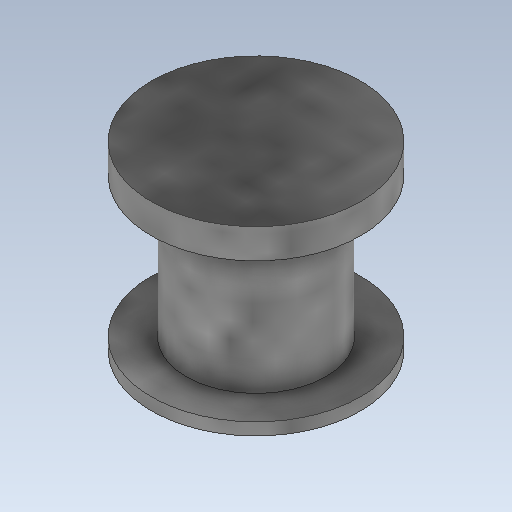
# Autodesk Inventor part: Wheel 75 mm - Part 5
Saved by Autodesk Inventor 2020 (Build 240168000, 168)
## iProperties
Created: 2022-11-14
Part Number: Wheel 75 mm - Part 5
Material: Generic
Document SubType Name: Modeling
Designer: saad.nashed
Density: 1 g/cm^3
Appearance: Steel Galvanized
Author: saad.nashed
Autodesk Inventor part; units mm, degrees
ref_plane "YZ Plane" through (0, 0, 0) normal (1, 0, 0) x (0, 1, 0)
ref_plane "XZ Plane" through (0, 0, 0) normal (0, 1, 0) x (-1, 0, 0)
ref_plane "XY Plane" through (0, 0, 0) normal (0, 0, 1) x (1, 0, 0)
sketch "Sketch1" plane through (0, 0, 0) normal (0, 0, 1) x (1, 0, 0)
  line L0 (0, 0) -> (0, 11.4)
  line L1 (0, 11.4) -> (6, 11.4)
  line L2 (6, 11.4) -> (6, 9.7)
  line L3 (6, 9.7) -> (4, 9.7)
  line L4 (4, 9.7) -> (4, 1.7)
  line L5 (4, 1.7) -> (6, 1.7)
  line L6 (6, 1.7) -> (6, 1)
  line L7 (4, 0) -> (0, 0)
  line L8 (6, 1) -> (4, 0)
  point P0 (6, 0)
  dimension "d0" = 8
  dimension "d1" = 6
  dimension "d2" = 4
  dimension "d3" = 1.7
  dimension "d5" = 1.7
  dimension "d6" = 1
  dimension "d7" = 2
  constraints: 18 end point, 6 perpendicular, 2 point on line, 1 vertical
  measures "d0" distance between parallel lines of L5 L3
  measures "d1" distance between parallel lines of L2 L0
  measures "d2" distance between parallel lines of L0 L4
  measures "d3" distance between parallel lines of L1 L3
  measures "d5" distance between parallel lines of L5 L7
  measures "d6" distance from line of L6.end L7
  measures "d7" distance from line of L7.start L6
revolve "Revolution1" add sketch "Sketch1" angle 360 about axis through (0, 0, 0) along (0, 1, 0)
sketch "Sketch2" plane through (0, 0, 0) normal (0, -1, 0) x (1, 0, 0)
  line L0 (0, 0) -> (3.4395, 12.8364)
  line L1 (3.4395, 12.8364) -> (-3.4395, 12.8364)
  line L2 (-3.4395, 12.8364) -> (0, 0)
  line L3 (0, 0) -> (0, -2.5884)
  dimension "d8" = 30
  constraints: 8 end point, 1 horizontal, 1 vertical, 1 other
  measures "d8" angle of L0 L2
extrude "Extrusion1" cut sketch "Sketch2" against normal blind 1.2 draft -60
pattern_circular "Circular Pattern1" count 6 over 360 about axis through (0, -10, 0) along (0, 1, 0) of "Extrusion1"
equation "\"d2\" = d25"
equation "\"d25\" = 4"
body "Solid1"
